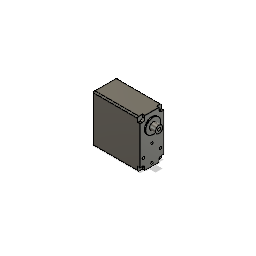
_main servo part.523e0f5b-3f12-431d-9e60-e8308424ebbb (Autodesk Fusion 360 design; units mm, degrees)
Autodesk Fusion 360 part; units mm, degrees
sketch "Sketch1" plane through (0, 0, 0) normal (1, 0, 0) x (0, 0, -1)
  line L0 (0, 0) -> (-20, 0)
  line L1 (-20, 0) -> (-20, 40)
  line L2 (-20, 40) -> (0, 40)
  line L3 (0, 40) -> (0, 0)
  dimension "d34" = 20
  dimension "d35" = 40
extrude "Extrude1" add sketch "Sketch1" along normal blind 40
sketch "Sketch2" plane through (40, 0, 0) normal (1, 0, 0) x (0, 0, -1)
  line L0 (0, 40) -> (-20, 40)
  line L1 (-20, 40) -> (-20, 0)
  line L2 (-20, 0) -> (0, 0)
  line L3 (0, 0) -> (0, 40)
  line L4 (-10, 40) -> (-10, 30) construction
  circle A0 centre (-10, 30) radius 6.25
  circle A1 centre (-10, 30) radius 3
  line L5 (-20, 0) -> (-20, 2.5) construction
  line L6 (-20, 2.5) -> (0, 2.5) construction
  line L7 (-20, 2.5) -> (-17.25, 2.5) construction
  line L8 (-17.25, 2.5) -> (-17.25, 41) construction
  line L9 (-17.25, 2.5) -> (-2.75, 2.5) construction
  line L10 (-2.75, 2.5) -> (-2.75, 37.5) construction
  line L11 (-2.75, 37.5) -> (-17.25, 37.5) construction
  line L12 (-17.25, 37.5) -> (-17.25, 2.5) construction
  line L13 (-17.25, 2.5) -> (-17.25, 17) construction
  line L14 (-17.25, 17) -> (-2.75, 17) construction
  circle A2 centre (-17.25, 17) radius 1
  circle A3 centre (-2.75, 17) radius 1
  circle A4 centre (-2.75, 2.5) radius 1
  circle A5 centre (-17.25, 2.5) radius 1
  circle A6 centre (-17.25, 37.5) radius 1
  circle A7 centre (-2.75, 37.5) radius 1
  dimension "d38" = 10
  dimension "d39" = 12.5
  dimension "d40" = 6
  dimension "d45" = 2.5
  dimension "d46" = 20
  dimension "d48" = 2.75
  dimension "d49" = 38.5
  dimension "d50" = 14.5
  dimension "d51" = 35
  dimension "d52" = 14.5
  dimension "d53" = 2
  dimension "d54" = 2
  dimension "d55" = 2
  dimension "d56" = 2
  dimension "d57" = 2
  dimension "d58" = 2
  measures "d39" diameter of A0
  measures "d40" diameter of A1
  measures "d45" distance of L2.end
  measures "d53" diameter of A2
  measures "d54" diameter of A3
  measures "d55" diameter of A4
  measures "d56" diameter of A5
  measures "d57" diameter of A6
  measures "d58" diameter of A7
extrude "Extrude4" cut sketch "Sketch2" against normal blind 5 contours A2 | A3 | A4 | A5 | A6 | A7
extrude "Extrude3" add sketch "Sketch2" along normal blind 1 contours A0
extrude "Extrude2" add sketch "Sketch2" along normal blind 4.5 contours A1
fillet "Fillet1" radius 1 4 edges at (40, 20, 20) (40, 40, 10) (40, 20, 0) (40, 0, 10)
sketch "Sketch3" plane through (0, 0, 0) normal (-1, 0, 0) x (0, 0, 1)
  line L0 (20, 40) -> (0, 40)
  line L1 (0, 40) -> (0, 0)
  line L2 (0, 0) -> (20, 0)
  line L3 (20, 0) -> (20, 40)
  circle A0 centre (10, 30) radius 6.25
  circle A1 centre (10, 30) radius 3
  dimension "d62" = 12.5
  dimension "d63" = 6
  measures "d62" diameter of A0
  measures "d63" diameter of A1
extrude "Extrude5" add sketch "Sketch3" along normal blind 6 contours A1
extrude "Extrude6" add sketch "Sketch3" along normal blind 1 contours A0
fillet "Fillet2" radius 1 2 edges at (19.5, 40, 20) (39.7071, 39.7071, 19.7071)
fillet "Fillet3" radius 1 2 edges at (19.5, 40, 0) (39.7071, 39.7071, 0.2929)
fillet "Fillet4" radius 1 2 edges at (19.5, 0, 20) (39.7071, 0.2929, 19.7071)
fillet "Fillet5" radius 1 2 edges at (19.5, 0, 0) (39.7071, 0.2929, 0.2929)
sketch "Sketch4" plane through (0, 0, 0) normal (-1, 0, 0) x (0, 0, 1)
  circle A0 centre (10, 30) radius 6.25
  arc A1 (0, 1) -> (1, 0) centre (1, 1) ccw
  line L0 (1, 0) -> (19, 0)
  arc A2 (19, 0) -> (20, 1) centre (19, 1) ccw
  line L1 (20, 1) -> (20, 39)
  arc A3 (20, 39) -> (19, 40) centre (19, 39) ccw
  line L2 (19, 40) -> (1, 40)
  arc A4 (1, 40) -> (0, 39) centre (1, 39) ccw
  line L3 (0, 39) -> (0, 1)
  line L4 (0, 0) -> (4, 0)
  line L5 (4, 0) -> (4, 4)
  line L6 (4, 4) -> (0, 4)
  line L7 (0, 4) -> (0, 0)
  line L8 (20, 0) -> (16, 0)
  line L9 (16, 0) -> (16, 4)
  line L10 (16, 4) -> (20, 4)
  line L11 (20, 4) -> (20, 0)
  line L12 (20, 40) -> (16, 40)
  line L13 (16, 40) -> (16, 36)
  line L14 (16, 36) -> (20, 36)
  line L15 (20, 36) -> (20, 40)
  line L16 (0, 40) -> (4, 40)
  line L17 (4, 40) -> (4, 36)
  line L18 (4, 36) -> (0, 36)
  line L19 (0, 36) -> (0, 40)
  dimension "d72" = 4
  dimension "d73" = 4
  dimension "d77" = 4
  dimension "d78" = 4
  dimension "d79" = 4
  dimension "d80" = 4
  dimension "d81" = 4
  dimension "d82" = 4
  measures "d72" distance of L4.start
  measures "d73" distance of L4.start
  measures "d79" distance of L4.start
  measures "d81" distance of L4.start
extrude "Extrude8" cut sketch "Sketch4" against normal blind 2 contours L2 A4 L3 L16 L17 L18 L19 | L0 A2 L1 L8 L9 L10 L11 | L1 A3 L2 L12 L13 L14 L15
extrude "Extrude7" cut sketch "Sketch4" against normal blind 2 contours A1 L0 L3 L4 L5 L6 L7
fillet "Fillet6" radius 2 1 edges at (1, 4, 4)
fillet "Fillet7" radius 2 1 edges at (1, 4, 16)
fillet "Fillet8" radius 2 1 edges at (1, 36, 16)
fillet "Fillet9" radius 2 1 edges at (1, 36, 4)
move_body "Move1" bodies 1 to x (1, 0, 0) y (0, 1, 0) z (0, 0, 1) at (-20, 0, -10)
move_body "Move2" bodies 1 to x (-1, 0, 0) y (0, 1, 0) z (0, 0, -1) at (-38, 0, -18)
move_body "Move3" bodies 1 to x (1, 0, 0) y (0, 1, 0) z (0, 0, 1) at (38.0076, 4, 17.9164)
sketch "Sketch5" plane through (20.0076, 0, 0) normal (1, 0, 0) x (0, 0, -1)
  circle A0 centre (0.0836, 34) radius 6.25
  line L0 (-9.9164, 8) -> (-7.9164, 8)
  arc A1 (-5.9164, 6) -> (-7.9164, 8) centre (-7.9164, 6) ccw
  line L1 (-5.9164, 6) -> (-5.9164, 4)
  line L2 (-5.9164, 4) -> (6.0836, 4)
  line L3 (6.0836, 4) -> (6.0836, 6)
  arc A2 (8.0836, 8) -> (6.0836, 6) centre (8.0836, 6) ccw
  line L4 (8.0836, 8) -> (10.0836, 8)
  line L5 (10.0836, 8) -> (10.0836, 40)
  line L6 (10.0836, 40) -> (8.0836, 40)
  arc A3 (6.0836, 42) -> (8.0836, 40) centre (8.0836, 42) ccw
  line L7 (6.0836, 42) -> (6.0836, 44)
  line L8 (6.0836, 44) -> (-5.9164, 44)
  line L9 (-5.9164, 44) -> (-5.9164, 42)
  arc A4 (-7.9164, 40) -> (-5.9164, 42) centre (-7.9164, 42) ccw
  line L10 (-7.9164, 40) -> (-9.9164, 40)
  line L11 (-9.9164, 40) -> (-9.9164, 8)
  circle A5 centre (0.0788, 13.7685) radius 4
  circle A6 centre (0.0788, 13.7685) radius 4
  circle A7 centre (0.0788, 13.7685) radius 4
  circle A8 centre (0.0788, 13.7685) radius 4
  circle A9 centre (0.0788, 13.7685) radius 4
  line L12 (0.0788, 13.7685) -> (-0.1, 13.7685)
  circle A10 centre (7.2788, 13.7522) radius 1
  circle A11 centre (7.2788, 13.7522) radius 1
  circle A12 centre (7.2788, 13.7522) radius 1
  circle A13 centre (7.2788, 13.7522) radius 1
  circle A14 centre (0.0788, 13.7685) radius 7.2 construction
  circle A15 centre (0.071, 6.5685) radius 1
  circle A16 centre (0.071, 6.5685) radius 1
  circle A17 centre (0.071, 6.5685) radius 1
  circle A18 centre (0.071, 6.5685) radius 1
  circle A19 centre (0.071, 6.5685) radius 1
  circle A20 centre (-7.1212, 13.752) radius 1
  circle A21 centre (-7.1212, 13.752) radius 1
  circle A22 centre (-7.1212, 13.752) radius 1
  circle A23 centre (-7.1212, 13.752) radius 1
  circle A24 centre (0.1328, 20.9683) radius 1
  circle A25 centre (0.1328, 20.9683) radius 1
  circle A26 centre (0.1328, 20.9683) radius 1
  circle A27 centre (0.1328, 20.9683) radius 1
  circle A28 centre (0.1328, 20.9683) radius 1
extrude "Extrude9" cut sketch "Sketch5" against normal blind 4 contours A10 A11 A12 A13 | A15 A16 A17 A18 A19 | A20 A21 A22 A23 | A24 A25 A26 A27 A28
sketch "Sketch6" plane through (26.0076, 0, 0) normal (1, 0, 0) x (0, 0, -1)
  circle A0 centre (0.0836, 34) radius 3
  circle A1 centre (0.0836, 34) radius 1.25
  dimension "d96" = 2.5
  measures "d96" diameter of A1
extrude "Extrude10" cut sketch "Sketch6" against normal blind 5 contours A1
sketch "Sketch7" plane through (0, 0, 0) normal (0, 0, 1) x (1, 0, 0)
sketch "Sketch8" plane through (20.0076, 0, 0) normal (1, 0, 0) x (0, 0, -1)
  circle A0 centre (0.1328, 20.9683) radius 1
  circle A1 centre (7.2788, 13.7522) radius 1
  circle A2 centre (-7.1212, 13.752) radius 1
  circle A3 centre (0.071, 6.5685) radius 1
  circle A4 centre (0.0836, 34) radius 6.25
  line L0 (-9.9164, 8) -> (-7.9164, 8)
  arc A5 (-5.9164, 6) -> (-7.9164, 8) centre (-7.9164, 6) ccw
  line L1 (-5.9164, 6) -> (-5.9164, 4)
  line L2 (-5.9164, 4) -> (6.0836, 4)
  line L3 (6.0836, 4) -> (6.0836, 6)
  arc A6 (8.0836, 8) -> (6.0836, 6) centre (8.0836, 6) ccw
  line L4 (8.0836, 8) -> (10.0836, 8)
  line L5 (10.0836, 8) -> (10.0836, 40)
  line L6 (10.0836, 40) -> (8.0836, 40)
  arc A7 (6.0836, 42) -> (8.0836, 40) centre (8.0836, 42) ccw
  line L7 (6.0836, 42) -> (6.0836, 44)
  line L8 (6.0836, 44) -> (-5.9164, 44)
  line L9 (-5.9164, 44) -> (-5.9164, 42)
  arc A8 (-7.9164, 40) -> (-5.9164, 42) centre (-7.9164, 42) ccw
  line L10 (-7.9164, 40) -> (-9.9164, 40)
  line L11 (-9.9164, 40) -> (-9.9164, 8)
sketch "Sketch9" plane through (0, 0, 0) normal (0, 1, 0) x (1, 0, 0)
sketch "Sketch10" plane through (20.1976, 7.5365, 20.8386) normal (1, 0, 0) x (0, 0, -1)
sketch "Sketch11" plane through (18.0076, 0, 0) normal (1, 0, 0) x (0, 0, -1)
  arc A0 (8.0836, 8) -> (6.0836, 6) centre (8.0836, 6) ccw
  line L0 (6.0836, 6) -> (6.0836, 4)
  line L1 (6.0836, 4) -> (9.0836, 4)
  arc A1 (9.0836, 4) -> (10.0836, 5) centre (9.0836, 5) ccw
  line L2 (10.0836, 5) -> (10.0836, 8)
  line L3 (10.0836, 8) -> (8.0836, 8)
  circle A2 centre (8.0836, 6) radius 2
